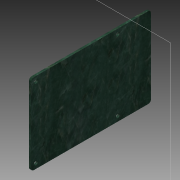
# Autodesk Inventor part: Bord
Saved by Autodesk Inventor 2015 (Build 190159000, 159)
## iProperties
Created: 2015-12-03
Part Number: Bord
Material: Generic
Document SubType Name: Modeling
Designer: david
Density: 1 g/cm^3
Appearance: Green Polished
Author: david
Autodesk Inventor part; units mm, degrees
ref_plane "YZ Plane" through (0, 0, 0) normal (1, 0, 0) x (0, 1, 0)
ref_plane "XZ Plane" through (0, 0, 0) normal (0, 1, 0) x (-1, 0, 0)
ref_plane "XY Plane" through (0, 0, 0) normal (0, 0, 1) x (1, 0, 0)
sketch "Sketch1" plane through (0, 0, 0) normal (1, 0, 0) x (0, 1, 0)
  line L0 (-40.5, 28.25) -> (40.5, 28.25)
  line L1 (42.5, 26.25) -> (42.5, -26.25)
  line L2 (40.5, -28.25) -> (-40.5, -28.25)
  line L3 (-42.5, -26.25) -> (-42.5, 26.25)
  line L4 (-42.5, 28.25) -> (42.5, -28.25) construction
  line L5 (42.5, 28.25) -> (-42.5, -28.25) construction
  arc A0 (40.5, -28.25) -> (42.5, -26.25) centre (40.5, -26.25) ccw
  arc A1 (42.5, 26.25) -> (40.5, 28.25) centre (40.5, 26.25) ccw
  arc A2 (-40.5, 28.25) -> (-42.5, 26.25) centre (-40.5, 26.25) ccw
  arc A3 (-42.5, -26.25) -> (-40.5, -28.25) centre (-40.5, -26.25) ccw
  point P0 (0, 0)
  dimension "d0" = 85
  dimension "d1" = 56.5
  dimension "d2" = 2
  constraints: 12 end point, 8 point on circle, 8 point on line, 8 tangent, 4 centre point, 3 equal radius, 2 midpoint, 2 parallel, 1 horizontal, 1 perpendicular
  measures "d0" distance of L4.end L5.end
  measures "d1" distance of L5.start L4.end
  measures "d2" radius of A0
extrude "Extrusion1" add sketch "Sketch1" along normal blind 1.5
sketch "Sketch2" plane through (0, 0, 0) normal (-1, 0, 0) x (0, 0, 1)
  circle A0 centre (-24.75, -39) radius 1.375
  line L0 (-26.25, -42.5) -> (26.25, -42.5) projected
  line L1 (-28.25, 40.5) -> (-28.25, -40.5) projected
  circle A1 centre (-24.75, 19) radius 1.375
  circle A2 centre (24.75, 19) radius 1.375
  circle A3 centre (24.75, -39) radius 1.375
  line L2 (28.25, -40.5) -> (28.25, 40.5) projected
  point P0 (0, 0)
  dimension "d5" = 2.75
  dimension "d6" = 3.5
  dimension "d7" = 3.5
  dimension "d8" = 2.75
  dimension "d9" = 2.75
  dimension "d10" = 2.75
  dimension "d11" = 3.5
  dimension "d12" = 58
  dimension "d13" = 58
  dimension "d14" = 3.5
  dimension "d15" = 3.5
  dimension "d16" = 3.5
  constraints: 4 centre point
  measures "d5" diameter of A0
  measures "d6" distance from line of L0 A0.centre
  measures "d7" distance from line of L1 A0.centre
  measures "d8" diameter of A1
  measures "d9" diameter of A2
  measures "d10" diameter of A3
  measures "d11" distance from line of L0 A3.centre
  measures "d12" distance of A2.centre A3.centre
  measures "d13" distance of A0.centre A1.centre
  measures "d14" distance from line of L2 A3.centre
  measures "d15" distance from line of L2 A2.centre
  measures "d16" distance from line of L1 A1.centre
extrude "Extrusion2" cut sketch "Sketch2" against normal blind 1.5
body "Solid1"
